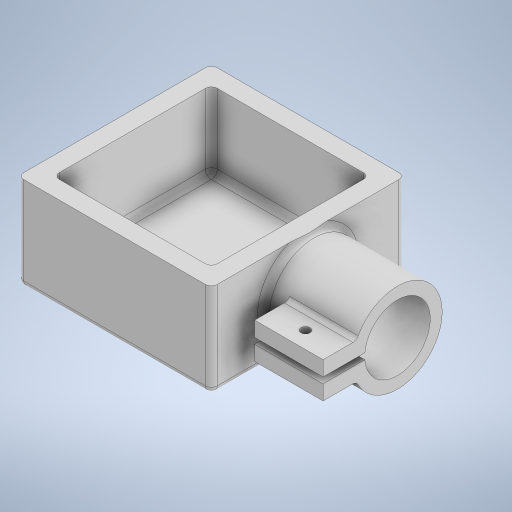
# Autodesk Inventor part: joystickBOX
Saved by Autodesk Inventor 2023 (Build 270158000, 158)
## iProperties
Created: 2023-09-25
Part Number: joystickBOX
Material: Generic
Document SubType Name: Modeling
Designer: Nikita
Density: 1 g/cm^3
Appearance: Default
Author: Nikita
Autodesk Inventor part; units mm, degrees
ref_plane "YZ Plane" through (0, 0, 0) normal (1, 0, 0) x (0, 1, 0)
ref_plane "XZ Plane" through (0, 0, 0) normal (0, 1, 0) x (-1, 0, 0)
ref_plane "XY Plane" through (0, 0, 0) normal (0, 0, 1) x (1, 0, 0)
sketch "Sketch1" plane through (0, 0, 0) normal (0, 1, 0) x (-1, 0, 0)
  line L0 (0, 0) -> (0, -65)
  line L1 (0, -65) -> (65, -65)
  line L2 (65, -65) -> (65, 0)
  line L3 (65, 0) -> (0, 0)
  dimension "d0" = 65
  dimension "d1" = 65
  dimension "d2" = 65
  constraints: 8 end point, 2 vertical, 1 perpendicular
  measures "d0" distance of L0.start L0.end
  measures "d1" distance of L0.end L1.end
  measures "d2" distance of L1.end L2.end
extrude "Extrusion1" add sketch "Sketch1" along normal blind 6
sketch "Sketch2" plane through (0, 6, 0) normal (0, 1, 0) x (1, 0, 0)
  line L0 (-65, 65) -> (-65, 0) projected
  line L1 (-65, 0) -> (-65, 6)
  line L2 (-59, 6) -> (-6, 6)
  line L3 (-6, 6) -> (-6, 59)
  line L4 (-6, 59) -> (-59, 59)
  line L5 (-59, 59) -> (-59, 6)
  line L6 (-65, 0) -> (0, 0) projected
  line L7 (-65, 0) -> (0, 0)
  line L8 (0, 0) -> (0, 65) projected
  line L9 (0, 0) -> (0, 65)
  line L10 (0, 65) -> (-65, 65) projected
  line L11 (0, 65) -> (-65, 65)
  line L12 (-65, 65) -> (-65, 0)
  dimension "d5" = 6
  constraints: 18 end point, 4 perpendicular, 1 collinear, 1 horizontal, 1 point on line
  measures "d5" distance of L0.end L1.end
extrude "Extrusion2" add sketch "Sketch2" along normal blind 25.5
sketch "Sketch3" plane through (0, 0, 0) normal (1, 0, 0) x (0, 0, -1)
  line L0 (0, 31.5) -> (65, 31.5) projected
  line L1 (65, 0) -> (65, 31.5) projected
  line L2 (65, 0) -> (0, 0) projected
  circle A0 centre (32.5, 15.75) radius 11
  circle A1 centre (32.5, 15.75) radius 15
  dimension "d11" = 22
  dimension "d12" = 30
  constraints: 2 centre point, 1 coincident
  measures "d11" diameter of A0
  measures "d12" diameter of A1
extrude "Extrusion3" add sketch "Sketch3" along normal blind 30
sketch "Sketch4" plane through (0, 15.75, -32.5) normal (1, 0, 0) x (0, 0, -1)
  circle A0 centre (0, 0) radius 11
  point P0 (-32.5, -15.75)
  constraints: 1 centre point
extrude "Extrusion4" cut sketch "Sketch4" against normal blind 6.25
fillet "Fillet1" radius 2 1 edges at (-59, 18.75, -59)
fillet "Fillet2" radius 2 1 edges at (-32.5, 0, 0)
fillet "Fillet3" radius 2 3 edges at (0, 0.5858, -0.5858) (0, 16.75, 0) (0, 0, -33.5)
fillet "Fillet4" radius 2 3 edges at (-65, 0.5858, -0.5858) (-65, 0, -33.5) (-65, 16.75, 0)
fillet "Fillet5" radius 2 5 edges at (-32.5, 0, -65) (-0.5858, 0.5858, -65) (0, 16.75, -65) (-65, 16.75, -65) (-64.4142, 0.5858, -65)
fillet "Fillet6" radius 2 1 edges at (-6, 18.75, -59)
fillet "Fillet7" radius 2 1 edges at (-6, 18.75, -6)
fillet "Fillet8" radius 2 3 edges at (-0.4388, 0.75, -32.5) (0, 7.5318, -45.0483) (0, 28.2983, -24.2818)
fillet "Fillet9" radius 2 2 edges at (-6, 25.158, -26.8001) (-6, 10.0501, -41.908)
fillet "Fillet10" radius 2 1 edges at (-59, 18.75, -6)
fillet "Fillet11" radius 2 11 edges at (-58.4142, 6, -6.5858) (-32.5, 6, -6) (-6.5858, 6, -6.5858) (-6, 6, -15.9507) (-5.5182, 6, -26.0361) (-58.4142, 6, -58.4142) (-32.5, 6, -59) (-6.5858, 6, -58.4142) (-6, 6, -49.0493) (-5.5182, 6, -38.9639) (-59, 6, -32.5)
sketch "Sketch5" plane through (30, 15.75, -32.5) normal (1, 0, 0) x (0, 0, -1)
  line L0 (-11.0788, 0.0781) -> (-11.0788, 1.0781)
  line L1 (-11.0788, 1.0781) -> (-15.0509, 1.0781)
  line L2 (-15.0509, 1.0781) -> (-15.0509, -0.9219)
  line L3 (-15.0509, -0.9219) -> (-10.9403, -0.9219)
  line L4 (-11.0788, 1.0781) -> (-10.5523, 1.0781)
  line L5 (-10.5523, 1.0781) -> (-10.5523, -0.9219)
  line L6 (-10.5523, -0.9219) -> (-10.9087, -0.9219)
  line L7 (-10.9087, -0.9219) -> (-10.9403, -0.9219)
  point P0 (-32.5, -15.75)
  dimension "d28" = 1
  dimension "d29" = 2
  constraints: 16 end point, 4 perpendicular, 2 vertical, 1 collinear, 1 point on line
  measures "d28" distance of L0.start L0.end
  measures "d29" distance of L1.end L2.end
extrude "Extrusion5" cut sketch "Sketch5" against normal blind 23
sketch "Sketch6" plane through (30, 0, 0) normal (1, 0, 0) x (0, 0, -1)
  arc A0 (41.3208, 3.6176) -> (23.6792, 3.6176) centre (32.5, 15.75) ccw projected
  line L0 (17.5391, 16.833) -> (17.5391, 21.833)
  line L1 (17.5391, 21.833) -> (18.7888, 21.833)
  arc A1 (17.5388, 16.8281) -> (17.5284, 14.8281) centre (32.5, 15.75) ccw projected
  line L2 (18.7888, 21.833) -> (17.5388, 16.8281)
  point P0 (0, 0)
  dimension "d32" = 5
  constraints: 6 end point, 2 point on circle, 1 perpendicular, 1 vertical
  measures "d32" distance of L0.start L0.end
extrude "Extrusion6" add sketch "Sketch6" against normal blind 23 contours A0 L0 L1
sketch "Sketch7" plane through (30, 0, 0) normal (1, 0, 0) x (0, 0, -1)
  line L0 (21.5387, 14.8281) -> (17.5284, 14.8281) projected
  line L1 (17.5284, 14.8281) -> (17.5284, 9.8281)
  line L2 (17.5284, 9.8281) -> (18.7185, 9.8281)
  arc A0 (17.5284, 14.8281) -> (18.7888, 21.833) centre (32.5, 15.75) ccw projected
  line L3 (18.7185, 9.8281) -> (18.7185, 14.8281)
  line L4 (18.7185, 14.8281) -> (17.5284, 14.8281)
  point P0 (0, 0)
  dimension "d35" = 5
  constraints: 8 end point, 2 perpendicular, 2 vertical, 1 point on circle
  measures "d35" distance of L0.end L1.end
extrude "Extrusion7" add sketch "Sketch7" against normal blind 23
sketch "Sketch8" plane through (30, 16.833, -17.5391) normal (0, 0, 1) x (1, 0, 0)
  line L0 (-23, 5) -> (0, 5) projected
  line L1 (-23, 5) -> (-23, -0.0049)
  line L2 (0, 0) -> (-23, 0) projected
  line L3 (-23, -0.0049) -> (0, 0)
  line L4 (0, 0) -> (0, 5)
  line L5 (0, 9.917) -> (0, -12.083) projected
  line L6 (-23, 5) -> (0, 5)
  point P0 (-30, -16.833)
  point P1 (0, -0.0049)
  point P2 (0, -2.0049)
  constraints: 8 end point, 1 perpendicular, 1 point on line
extrude "Extrusion8" add sketch "Sketch8" along normal blind 10 contours L0 L4 L2 L1
sketch "Sketch9" plane through (30, 9.8281, -17.5284) normal (0, 0, 1) x (1, 0, 0)
  line L0 (-23, 0) -> (-23, 5) projected
  line L1 (-23, 5) -> (-23, 0)
  line L2 (-23, 0) -> (0, 0)
  line L3 (0, 5) -> (-23, 5) projected
  line L4 (0, 0) -> (0, 5)
  line L5 (0, 5) -> (-23, 5)
  point P0 (-30, -9.8281)
  constraints: 8 end point, 3 perpendicular, 1 vertical
extrude "Extrusion9" add sketch "Sketch9" along normal blind 10
sketch "Sketch10" plane through (7, 21.833, -18.7888) normal (0, 1, 0) x (1, 0, 0)
  line L0 (23, -0.0703) -> (0, -0.0703) construction
  line L1 (23, -11.2604) -> (23, -0.0703) construction
  line L2 (0, -0.0703) -> (23, -11.2604) construction
  line L3 (23, -11.2604) -> (23, -0.0703) construction
  line L4 (23, -0.0703) -> (0, -11.2604) construction
  circle A0 centre (11.5, -5.6654) radius 1.5
  point P0 (-7, -18.7888)
  dimension "d42" = 3
  constraints: 6 end point, 1 centre point, 1 midpoint, 1 vertical
  measures "d42" diameter of A0
extrude "Extrusion10" cut sketch "Sketch10" against normal blind 18.75
fillet "Fillet12" radius 2 1 edges at (18.5, 21.833, -18.7888)
fillet "Fillet13" radius 2 1 edges at (18.5, 9.8281, -18.7185)
body "Solid1"
